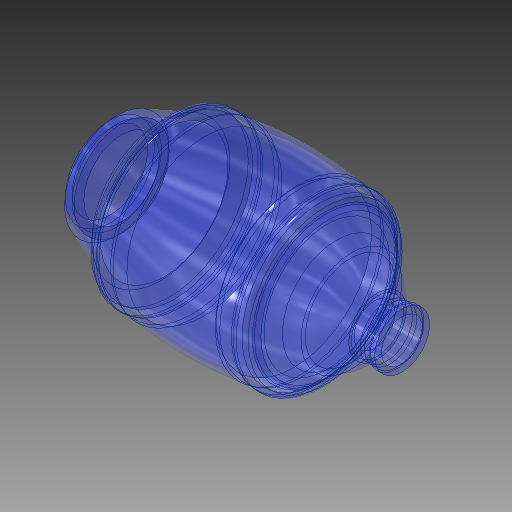
# Autodesk Inventor part: Corpo do Ambu
Saved by Autodesk Inventor 2019 (Build 230136000, 136)
## iProperties
Created: 2020-04-02
Part Number: Corpo do Ambu
Material: Genérico
Document SubType Name: Modeling
Designer: Paulo Rodrigues
Density: 1 g/cm^3
Appearance: Transparente - Azul
Author: Paulo Rodrigues
Autodesk Inventor part; units mm, degrees
ref_plane "YZ Plane" through (0, 0, 0) normal (1, 0, 0) x (0, 1, 0)
ref_plane "XZ Plane" through (0, 0, 0) normal (0, 1, 0) x (-1, 0, 0)
ref_plane "XY Plane" through (0, 0, 0) normal (0, 0, 1) x (1, 0, 0)
sketch "Esboço1" plane through (0, 0, 0) normal (0, 0, 1) x (1, 0, 0)
  line L0 (-39, 0) -> (39, 0)
  arc A0 (37.3328, 60.4247) -> (-37.3328, 60.4247) centre (0, -89.6) ccw
  arc A1 (-48.2727, 59.7222) -> (-39.7942, 59.6991) centre (-44, 72) ccw
  arc A2 (39.7942, 59.6991) -> (48.2727, 59.7222) centre (44, 72) ccw
  line L1 (-49.9161, 60) -> (-52, 60)
  line L2 (-57, 55) -> (-57, 53.8775)
  line L3 (49.9161, 60) -> (52, 60)
  line L4 (57, 55) -> (57, 53.1664)
  line L5 (-39, 0) -> (-111.5885, 0)
  line L6 (-95, 38) -> (-95, 32.5)
  line L7 (-95, 38) -> (-58.287, 52.0089)
  line L8 (-95, 32.5) -> (-100, 32.5)
  line L9 (95, 21) -> (95, 19)
  arc A3 (57.4077, 51.9562) -> (76, 36.75) centre (98.4128, 83.123) ccw
  arc A4 (95, 21) -> (76, 36.75) centre (53.5872, -9.623) ccw
  line L10 (113, 19) -> (113, 15)
  line L11 (113, 15) -> (113, 20)
  line L12 (113, 20) -> (109, 20)
  line L13 (109, 20) -> (109, 19)
  arc A5 (101.5773, 19) -> (104.5724, 19) centre (103.0748, 19) ccw
  line L14 (95, 19) -> (101.5773, 19)
  line L15 (104.5724, 19) -> (109, 19)
  arc A6 (-52, 60) -> (-57, 55) centre (-52, 55) ccw
  arc A7 (57, 55) -> (52, 60) centre (52, 55) ccw
  arc A8 (-58.287, 52.0089) -> (-57, 53.8775) centre (-59, 53.8775) ccw
  arc A9 (57, 53.1664) -> (57.4077, 51.9562) centre (59, 53.1664) ccw
  line L16 (-100, 27.4953) -> (-91.4686, 27.4953)
  line L17 (-91.4686, 27.4953) -> (-91.4686, 34.6774)
  line L18 (-91.4686, 34.6774) -> (-41.5843, 53.75)
  line L19 (58.1587, 45.8187) -> (92.9264, 15)
  line L20 (92.9264, 15) -> (113, 15)
  arc A10 (42.8385, 54.2818) -> (-41.5843, 53.75) centre (1.5168, -87.2147) ccw
  arc A11 (58.1587, 45.8187) -> (42.8385, 54.2818) centre (31.6255, 15.8856) ccw
  line L21 (-100, 32.5) -> (-100, 27.4953)
  arc A12 (49.9161, 60) -> (48.2727, 59.7222) centre (49.9161, 55) ccw
  arc A13 (39.7942, 59.6991) -> (37.3328, 60.4247) centre (30.0884, 31.3126) ccw
  arc A14 (-37.3328, 60.4247) -> (-39.7942, 59.6991) centre (-30.0884, 31.3126) ccw
  arc A15 (-48.2727, 59.7222) -> (-49.9161, 60) centre (-49.9161, 55) ccw
  point P0 (0, 0)
  point P1 (-49, 60)
  point P2 (49, 60)
  point P3 (-57, 52.5)
  point P4 (57, 52.5)
  point P5 (52, 51.2779)
  dimension "d8" = 57
  dimension "d9" = 57
  dimension "d11" = 38
  dimension "d13" = 76
  dimension "d14" = 65
  dimension "d16" = 105
  dimension "d17" = 42
  dimension "d18" = 38
  dimension "d19" = 105
  dimension "d23" = 18
  dimension "d24" = 40
  dimension "d25" = 4
  dimension "d26" = 5
  dimension "d27" = 2
  dimension "d28" = 40
  dimension "d29" = 30
  dimension "d30" = 5
  dimension "d31" = 30
  dimension "d32" = 5
  constraints: 44 end point, 36 point on circle, 19 tangent, 16 centre point, 8 horizontal, 7 point on line, 4 perpendicular, 3 equal radius, 3 vertical, 2 parallel
  measures "d8" distance from line of L4 point (0, 0)
  measures "d9" distance from line of L2 point (0, 0)
  measures "d11" distance between parallel lines of L6 L2
  measures "d13" diameter of L6.start L5
  measures "d14" diameter of L8 L5
  measures "d16" diameter of point (-57, 52.5) L5
  measures "d17" diameter of L9.start L5
  measures "d18" distance between parallel lines of L9 L4
  measures "d19" diameter of point (57, 52.5) L5
  measures "d23" distance from line of L9 L10.start
  measures "d24" diameter of L12 L5
  measures "d25" distance between parallel lines of L11 L13
  measures "d26" radius of A6
  measures "d27" radius of A8
  measures "d28" radius of A11
  measures "d29" diameter of L20 L5
  measures "d30" radius of A12
  measures "d31" radius of A13
  measures "d32" radius of A15
revolve "Revolução1" add sketch "Esboço1" angle 360 about axis through (-39, 0, 0) along (-1, 0, 0)
sketch "Esboço2" plane through (0, 0, 0) normal (0, 1, 0) x (-1, 0, 0)
  arc A0 (48.2727, -59.7222) -> (39.7942, -59.6991) centre (44, -72) ccw projected
  line L0 (57, 55) -> (57, -55) projected
  line L1 (57, 55) -> (57, -55) projected
  line L2 (52, 60) -> (52, -60) projected
  arc A1 (58.287, -52.0089) -> (57, -53.8775) centre (59, -53.8775) ccw projected
  line L3 (95, -38) -> (58.287, -52.0089) projected
  line L4 (-39.7942, 59.6991) -> (-39.7942, -59.6991) projected
  line L5 (-48.2727, 59.7222) -> (-48.2727, -59.7222) projected
  arc A2 (-39.7942, -59.6991) -> (-48.2727, -59.7222) centre (-44, -72) ccw projected
  line L6 (-52, 60) -> (-52, -60) projected
  line L7 (-57, 55) -> (-57, -55) projected
  arc A3 (-57.4077, -51.9562) -> (-76, -36.75) centre (-98.4128, -83.123) ccw projected
  arc A4 (-57, -55) -> (-52, -60) centre (-52, -55) ccw projected
  arc A5 (-39.7942, -59.6991) -> (-48.2727, -59.7222) centre (-43.957, -87.7934) ccw
  arc A6 (48.2727, -59.7222) -> (39.7942, -59.6991) centre (43.9217, -100.7696) ccw
  arc A7 (52, -60) -> (57, -55) centre (52, -55) ccw projected
  arc A8 (62.8894, -50.2527) -> (56.4459, -57.2877) centre (75.2097, -68.0054) ccw
  arc A9 (-56.876, -56.1064) -> (-59.4688, -49.4162) centre (-80.8296, -61.5418) ccw
  line L8 (0, 0) -> (133.2313, 0)
  arc A10 (48.2727, -59.7222) -> (39.7942, -59.6991) centre (44, -72) ccw
  line L9 (62.8894, -50.2527) -> (58.287, -52.0089)
  arc A11 (58.287, -52.0089) -> (57, -53.8775) centre (59, -53.8775) ccw
  line L10 (57, -53.8775) -> (57, -55)
  arc A12 (56.4459, -57.2877) -> (57, -55) centre (52, -55) ccw
  line L11 (-39.7942, 59.6991) -> (-39.7942, -59.6991) projected
  arc A13 (-39.7942, -59.6991) -> (-48.2727, -59.7222) centre (-44, -72) ccw
  line L12 (-57, 53.1664) -> (-57, -53.1664) projected
  line L13 (-57.4077, 51.9562) -> (-57.4077, -51.9562) projected
  line L14 (-59.4688, -49.4162) -> (-57.4077, -51.9562)
  line L15 (-57, 53.1664) -> (-57, -53.1664) projected
  arc A14 (-57, -53.1664) -> (-57.4077, -51.9562) centre (-59.1237, -53.2081) ccw
  line L16 (-57, -53.1664) -> (-57, -55)
  line L17 (-57, 55) -> (-57, -55) projected
  arc A15 (-57, -55) -> (-56.876, -56.1064) centre (-52, -55) ccw
  constraints: 25 point on circle, 10 centre point, 10 end point, 4 concentric, 2 point on line, 1 collinear, 1 horizontal, 1 tangent, 1 vertical
revolve "Revolução2" add sketch "Esboço2" angle 360 about axis through (0, 0, 0) along (-1, 0, 0) contours A6 A0 | A1 L3 A8 A7 L0 | A5 A2 | L7 A4 A9 L14 A14
sketch "Esboço3" plane through (0, 0, 0) normal (0, 1, 0) x (-1, 0, 0)
  arc A0 (-37.3328, -60.4247) -> (37.3328, -60.4247) centre (0, 89.6) ccw projected
  arc A1 (-37.3328, -60.4247) -> (37.3328, -60.4247) centre (0, 212.1941) ccw
  arc A2 (-37.3328, -60.4247) -> (37.3328, -60.4247) centre (0, 89.6) ccw
  line L0 (0, 0) -> (155.1986, 0)
  constraints: 6 point on circle, 2 centre point, 2 end point, 1 concentric, 1 horizontal
revolve "Revolução3" cut sketch "Esboço3" angle 360 about axis through (0, 0, 0) along (-1, 0, 0)
sketch "Esboço4" plane through (0, 0, 0) normal (0, 0, 1) x (1, 0, 0)
  line L0 (-41.5843, -53.75) -> (-91.4686, -34.6774) projected
  arc A0 (-41.5843, -53.75) -> (42.8385, -54.2818) centre (1.5168, 87.2147) ccw projected
  arc A1 (42.8385, -54.2818) -> (58.1587, -45.8187) centre (31.6255, -15.8856) ccw projected
  line L1 (92.9264, -15) -> (58.1587, -45.8187) projected
  arc A2 (70.7276, -34.6774) -> (92.9264, -15) centre (61.2556, -1.6313) ccw
  line L2 (34.1111, -56.5433) -> (52.8578, -56.5433)
  line L3 (52.8578, -56.5433) -> (58.1587, -45.8187)
  line L4 (-31.0776, -56.5433) -> (-52.4928, -56.5433)
  line L5 (-52.4928, -56.5433) -> (-60.4206, -46.5482)
  line L6 (-60.4206, -46.5482) -> (-35.3119, -42.9158)
  line L7 (-35.3119, -42.9158) -> (-31.0776, -56.5433)
  line L8 (34.1111, -56.5433) -> (38.6643, -42.0466)
  line L9 (38.6643, -42.0466) -> (58.1587, -45.8187)
  line L10 (70.7276, -34.6774) -> (92.9264, -15)
  line L11 (0, 0) -> (-145.9148, 0)
  constraints: 20 end point, 6 point on circle, 4 point on line, 2 horizontal, 1 centre point, 1 collinear
revolve "Revolução4" cut sketch "Esboço4" angle 360 about axis through (0, 0, 0) along (-1, 0, 0) contours A0 L4 L5 L0 | A0 A1 L3 L2 | A2 L1
fillet "Arredondamento1" radius 40 2 edges at (70.7276, 0, -34.6774) (70.7276, 0, 34.6774)
equation "\"d9\" = d8"
